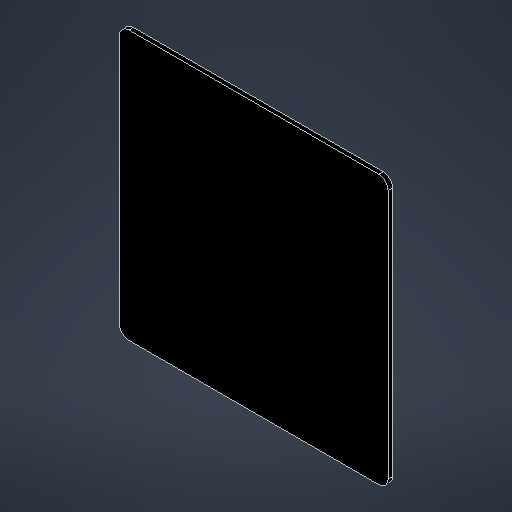
# Autodesk Inventor part: rv_ledbrick_8ch_BOARD
Saved by Autodesk Inventor 2026.1 (Build 301233020, 233B)
## iProperties
Created: 2025-09-11
Part Number: rv_ledbrick_8ch_BOARD
Material: Generic
Document SubType Name: Modeling
Designer: atrus
Density: 1 g/cm^3
Appearance: BoardColor
Author: atrus
Autodesk Inventor part; units mm, degrees
ref_plane "YZ Plane" through (0, 0, 0) normal (1, 0, 0) x (0, 1, 0)
ref_plane "XZ Plane" through (0, 0, 0) normal (0, 1, 0) x (-1, 0, 0)
ref_plane "XY Plane" through (0, 0, 0) normal (0, 0, 1) x (1, 0, 0)
ref_plane "BoardFrontPlane" through (0, 0, 0) normal (0, 0, 1) x (1, 0, 0)
sketch "Sketch1" plane through (0, 0, 0) normal (0, 0, 1) x (1, 0, 0)
  line L0 (30, 30) -> (30, 109)
  arc A0 (33, 112) -> (30, 109) centre (33, 109) ccw
  line L1 (33, 112) -> (112, 112)
  arc A1 (115, 109) -> (112, 112) centre (112, 109) ccw
  line L2 (115, 109) -> (115, 30)
  arc A2 (112, 27) -> (115, 30) centre (112, 30) ccw
  line L3 (112, 27) -> (33, 27)
  arc A3 (30, 30) -> (33, 27) centre (33, 30) ccw
  constraints: 8 end point, 8 point on circle, 4 centre point
extrude "BoardOutline" add sketch "Sketch1" along normal blind 1.4202
body "Solid1"
